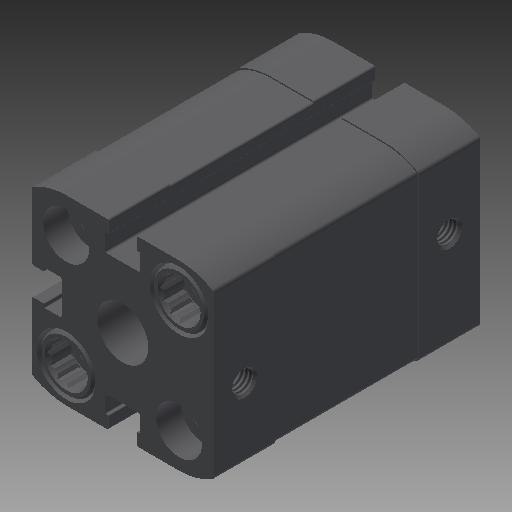
# Autodesk Inventor part: 536233 ADN-15-P---(Z)
Saved by Autodesk Inventor 2017 (Build 210142000, 142)
## iProperties
Category: PARTsolutions
Company: FESTO
Created: 2018-05-29
Part Number: 536233 ADN-15-P---(Z)
Catalog Web Link: www.cadenas.de
Description: ADN-(Z)-Compact cylinder - Z
Vendor: FESTO
Document SubType Name: Modeling
Designer: psAdmin
Manufacturer: FESTO
Mass: 44.5722 g
Surface Area: 191.377 cm^2
Volume: 44.5722 cm^3
Density: 1 g/cm^3
Material: Generic
Appearance: PSOLRGB-191-191-191
PSOL_IDENT_0: {$CADENAS_DATA\23d-libs\festo\parts\a\adn\parts\adn_zr.prj},210 {VTYP=3D},{NB=536233 ADN-15-P---(Z)}
PSOL_IDENT_1: ,{LINA=536233 ADN-15-P---(Z)},{NN=ADN-(Z)},{DATE=06.10.2015 11:54:02},{GEOMDATE=22.09.2015 09:31:00}
PSOL_IDENT_2: ,{VERSION=},{LINEID=8190},{LINESUBID=-1},{WBVAR=HUB,DF,Q,S2S20,S1,R8,TT}  {NB=536233 ADN-15-P---(Z)}
PSOL_IDENT_3: ,{LINA=536233 ADN-15-P---(Z)},{KT=536233},{TNR=536233},{AUSF=ADN},{KDM=20},{BG=19.500},{VERS=1},{HUB
PSOL_IDENT_4: P=-},{HUB=15.00000},{HUB1=[1-300]},{HUB2=[1-200]},{HUB3=0},{THC='A','I'},{DF=P},{GA=A},{HUBL=variabl
PSOL_IDENT_5: e},{HUBC=hubc error},{Q=-},{VAR1C='-','Q'},{S2S20=-},{VAR2C='-','S2','S20'},{VAR5C='-','S6'},{S1=-},
PSOL_IDENT_6: {R8=-},{R81='-','R8'},{TT=-},{TT1='-','TT'},{VAR6C='-'},{VAR7C='-','R3'},{HUBALG=[1-300]},{A=16.000}
PSOL_IDENT_7: ,{A1=0.000},{AF=14.000},{AF1=0.000},{AF2=12.000},{AF3=0.000},{B=0.000},{B1=18.000},{BG1=0.000},{D1=9
PSOL_IDENT_8: .000},{D2=9.000},{D3=4.100},{D4=0.000},{D5=6.000},{D6=M4},{D7=4.000},{D8=3.800},{D9=6.000},{E=35.500
PSOL_IDENT_9: },{EE=M5},{EEN=5.000},{EE1=-},{J=12.000},{J1=2.600},{J11=2.6},{J2=0.000},{KF=10-32 UNF-2B},{KF1=-},{
PSOL_IDENT_10: KF2=10-32 UNF-2B},{KF3=-},{KK=5/16-24 UNF-2A},{KK1=-},{L1=2.600},{L2=37.000},{L3=2.100},{L4=4.800},{
PSOL_IDENT_11: L5=0.000},{L6=51.000},{L7=17.000},{L8=2.000},{L9=2.000},{L10=0.000},{L11=0.000},{MF=8.000},{MM=10.00
PSOL_IDENT_12: 0},{MM1=0.000},{PL=6.000},{RT=M5},{RTN=5},{RTNK=4.134},{SF=11/32},{SF1=-},{SW=9.000},{TG=22.000},{VD=
PSOL_IDENT_13: 0.000},{VD1=5.200},{WH=5.700},{WH1=0.000},{WL=4.200},{WL1=0.000},{Y1=0.300},{Y2=0.500},{ZJ=42.700},{
PSOL_IDENT_14: ZM=48.400},{RU=23.800},{R1=12.750},{R2=0.800},{RA=0.000},{RB1=5.400},{RB2=6.800},{RT1=3.400},{DSK=8.
PSOL_IDENT_15: 000},{MDK=10.000},{MK=6.000},{MT=3.000},{MS=5.000},{RUB=0.400},{KFN=6.000},{KFK=4.917},{B111=11.500}
PSOL_IDENT_16: ,{B11=1.000},{B2=6.500},{B3=10.500},{B4=4.600},{B5=4.400},{B6=7.500},{B7=19.500},{B8=5.000},{B9=7.00
PSOL_IDENT_17: 0},{B10=8.400},{W=0.400},{S=7.000},{LA=0.000},{LA1=0.000},{LA2=5.500},{LA3=7.500},{LA31=11.000},{LA4=
PSOL_IDENT_18: 0.000},{LA5=0.000},{LA6=0.000},{RR=5.000},{LA7=0.000},{LA8=0.000},{LA9=0.000},{LA10=0.000},{ES=0.000
PSOL_IDENT_19: },{SS=0.000},{TS=0.000},{WS=0.000},{DK=0.000},{KS=0.000},{QN=},{S2N=},{S1S20N=},{R8N=},{TTN=},{DFALG='
PSOL_IDENT_20: P','PPS'}
NN: ADN-(Z)
NT: Compact cylinder - Z
NB: 536233 ADN-15-P---(Z)
NBSYN: $TNR. $AUSF.-$HUB.-$DF.$QN.$S2N.$S1S20N.$R8N.$TTN.---(Z)
LINA: 536233 ADN-15-P---(Z)
TNR: 536233
AUSF: ADN
KDM: 20
BG: 19.500
HUB: 15.00000
DF: P
GA: A
Q: -
S2S20: -
S1: -
R8: -
TT: -
A: 16.000
A1: 0.000
AF: 14.000
AF1: 0.000
AF2: 12.000
AF3: 0.000
B: 0.000
B1: 18.000
BG1: 0.000
D1: 9.000
D2: 9.000
D3: 4.100
D4: 0.000
D5: 6.000
D6: M4
D7: 4.000
D8: 3.800
D9: 6.000
E: 35.500
EE: M5
EE1: -
J: 12.000
J1: 2.600
J2: 0.000
KF: 10-32 UNF-2B
KF1: -
KF2: 10-32 UNF-2B
KF3: -
KK: 5/16-24 UNF-2A
KK1: -
L1: 2.600
L2: 37.000
L3: 2.100
L4: 4.800
L5: 0.000
L6: 51.000
L7: 17.000
L8: 2.000
L9: 2.000
L10: 0.000
L11: 0.000
MF: 8.000
MM: 10.000
MM1: 0.000
PL: 6.000
RT: M5
RTNK: 4.134
SF: 11/32
SF1: -
SW: 9.000
TG: 22.000
VD: 0.000
VD1: 5.200
WH: 5.700
WH1: 0.000
WL: 4.200
WL1: 0.000
Y1: 0.300
Y2: 0.500
ZJ: 42.700
ZM: 48.400
RU: 23.800
R1: 12.750
R2: 0.800
RA: 0.000
DSK: 8.000
MDK: 10.000
MK: 6.000
MT: 3.000
MS: 5.000
RUB: 0.400
B111: 11.500
B11: 1.000
B2: 6.500
B3: 10.500
B4: 4.600
B5: 4.400
B6: 7.500
B7: 19.500
B8: 5.000
B9: 7.000
B10: 8.400
W: 0.400
S: 7.000
LA: 0.000
LA1: 0.000
LA2: 5.500
LA3: 7.500
LA31: 11.000
LA4: 0.000
LA5: 0.000
LA6: 0.000
RR: 5.000
LA7: 0.000
LA8: 0.000
LA9: 0.000
LA10: 0.000
ES: 0.000
SS: 0.000
TS: 0.000
WS: 0.000
DK: 0.000
KS: 0.000
SUPPLIER: FESTO
ARTICLENO: 536233 ADN-15-P---(Z)
BOMINFO: 536233 ADN-15-P---(Z)
CREATOR: CADENAS GmbH
Title: 536233 ADN-15-P---(Z)
Author: Cadenas PARTsolutions
Comments: Compact cylinder - Z
Autodesk Inventor part; units mm, degrees
sketch "Skizze_1" plane through (0, 0, 0) normal (0, 0, 1) x (1, 0, 0)
  line L0 (-17.75, -3.1) -> (-17.75, -15.3634)
  arc A0 (-17.75, -15.3634) -> (-17.3483, -16.0572) centre (-16.95, -15.3634) ccw
  arc A1 (-17.3483, -16.0572) -> (-11, -17.75) centre (-11, -5) ccw
  line L1 (-11, -17.75) -> (-3.1, -17.75)
  arc A2 (-3.1, -17.75) -> (-2.7, -17.35) centre (-3.1, -17.35) ccw
  line L2 (-2.7, -17.35) -> (-2.7, -15.5)
  arc A3 (-2.7, -15.5) -> (-2.9, -15.3) centre (-2.9, -15.5) ccw
  line L3 (-2.9, -15.3) -> (-3.2, -15.3)
  arc A4 (-3.4, -15.1) -> (-3.2, -15.3) centre (-3.2, -15.1) ccw
  line L4 (-3.4, -15.1) -> (-3.4, -12.3)
  arc A5 (-3, -11.9) -> (-3.4, -12.3) centre (-3, -12.3) ccw
  line L5 (-3, -11.9) -> (3, -11.9)
  arc A6 (3.4, -12.3) -> (3, -11.9) centre (3, -12.3) ccw
  line L6 (3.4, -12.3) -> (3.4, -15.1)
  arc A7 (3.2, -15.3) -> (3.4, -15.1) centre (3.2, -15.1) ccw
  line L7 (3.2, -15.3) -> (2.9, -15.3)
  arc A8 (2.9, -15.3) -> (2.7, -15.5) centre (2.9, -15.5) ccw
  line L8 (2.7, -15.5) -> (2.7, -17.35)
  arc A9 (2.7, -17.35) -> (3.1, -17.75) centre (3.1, -17.35) ccw
  line L9 (3.1, -17.75) -> (11, -17.75)
  arc A10 (11, -17.75) -> (17.3483, -16.0572) centre (11, -5) ccw
  arc A11 (17.3483, -16.0572) -> (17.75, -15.3634) centre (16.95, -15.3634) ccw
  line L10 (17.75, -15.3634) -> (17.75, 15.3634)
  arc A12 (17.75, 15.3634) -> (17.3483, 16.0572) centre (16.95, 15.3634) ccw
  arc A13 (17.3483, 16.0572) -> (11, 17.75) centre (11, 5) ccw
  line L11 (11, 17.75) -> (3.1, 17.75)
  arc A14 (3.1, 17.75) -> (2.7, 17.35) centre (3.1, 17.35) ccw
  line L12 (2.7, 17.35) -> (2.7, 15.5)
  arc A15 (2.7, 15.5) -> (2.9, 15.3) centre (2.9, 15.5) ccw
  line L13 (2.9, 15.3) -> (3.2, 15.3)
  arc A16 (3.4, 15.1) -> (3.2, 15.3) centre (3.2, 15.1) ccw
  line L14 (3.4, 15.1) -> (3.4, 12.3)
  arc A17 (3, 11.9) -> (3.4, 12.3) centre (3, 12.3) ccw
  line L15 (3, 11.9) -> (-3, 11.9)
  arc A18 (-3.4, 12.3) -> (-3, 11.9) centre (-3, 12.3) ccw
  line L16 (-3.4, 12.3) -> (-3.4, 15.1)
  arc A19 (-3.2, 15.3) -> (-3.4, 15.1) centre (-3.2, 15.1) ccw
  line L17 (-3.2, 15.3) -> (-2.9, 15.3)
  arc A20 (-2.9, 15.3) -> (-2.7, 15.5) centre (-2.9, 15.5) ccw
  line L18 (-2.7, 15.5) -> (-2.7, 17.35)
  arc A21 (-2.7, 17.35) -> (-3.1, 17.75) centre (-3.1, 17.35) ccw
  line L19 (-3.1, 17.75) -> (-11, 17.75)
  arc A22 (-11, 17.75) -> (-17.3483, 16.0572) centre (-11, 5) ccw
  arc A23 (-17.3483, 16.0572) -> (-17.75, 15.3634) centre (-16.95, 15.3634) ccw
  line L20 (-17.75, 15.3634) -> (-17.75, 3.1)
  arc A24 (-17.75, 3.1) -> (-17.35, 2.7) centre (-17.35, 3.1) ccw
  line L21 (-17.35, 2.7) -> (-15.5, 2.7)
  arc A25 (-15.5, 2.7) -> (-15.3, 2.9) centre (-15.5, 2.9) ccw
  line L22 (-15.3, 2.9) -> (-15.3, 3.2)
  arc A26 (-15.1, 3.4) -> (-15.3, 3.2) centre (-15.1, 3.2) ccw
  line L23 (-15.1, 3.4) -> (-12.3, 3.4)
  arc A27 (-11.9, 3) -> (-12.3, 3.4) centre (-12.3, 3) ccw
  line L24 (-11.9, 3) -> (-11.9, -3)
  arc A28 (-12.3, -3.4) -> (-11.9, -3) centre (-12.3, -3) ccw
  line L25 (-12.3, -3.4) -> (-15.1, -3.4)
  arc A29 (-15.3, -3.2) -> (-15.1, -3.4) centre (-15.1, -3.2) ccw
  line L26 (-15.3, -3.2) -> (-15.3, -2.9)
  arc A30 (-15.3, -2.9) -> (-15.5, -2.7) centre (-15.5, -2.9) ccw
  line L27 (-15.5, -2.7) -> (-17.35, -2.7)
  arc A31 (-17.35, -2.7) -> (-17.75, -3.1) centre (-17.35, -3.1) ccw
  constraints: 64 point on circle, 56 end point, 32 centre point
extrude "Extrusion1" add sketch "Skizze_1" against normal blind 52
sketch "Sketch_111" plane through (0, 0, -12) normal (0, 0, 1) x (1, 0, 0)
  line L0 (-35.5, 35.5) -> (-35.5, -35.5)
  line L1 (-35.5, -35.5) -> (35.5, -35.5)
  line L2 (35.5, -35.5) -> (35.5, 35.5)
  line L3 (35.5, 35.5) -> (-35.5, 35.5)
  line L4 (-17.5, -3.1) -> (-17.5, -15.253)
  arc A0 (-17.5, -15.253) -> (-17.0816, -15.9561) centre (-16.7, -15.253) ccw
  arc A1 (-17.0816, -15.9561) -> (-11, -17.5) centre (-11, -4.75) ccw
  line L5 (-11, -17.5) -> (-3.1, -17.5)
  arc A2 (-3.1, -17.5) -> (-2.7, -17.1) centre (-3.1, -17.1) ccw
  line L6 (-2.7, -17.1) -> (-2.7, -15.45)
  arc A3 (-2.7, -15.45) -> (-2.85, -15.3) centre (-2.85, -15.45) ccw
  line L7 (-2.85, -15.3) -> (-3.2, -15.3)
  arc A4 (-3.4, -15.1) -> (-3.2, -15.3) centre (-3.2, -15.1) ccw
  line L8 (-3.4, -15.1) -> (-3.4, -12.3)
  arc A5 (-3, -11.9) -> (-3.4, -12.3) centre (-3, -12.3) ccw
  line L9 (-3, -11.9) -> (3, -11.9)
  arc A6 (3.4, -12.3) -> (3, -11.9) centre (3, -12.3) ccw
  line L10 (3.4, -12.3) -> (3.4, -15.1)
  arc A7 (3.2, -15.3) -> (3.4, -15.1) centre (3.2, -15.1) ccw
  line L11 (3.2, -15.3) -> (2.85, -15.3)
  arc A8 (2.85, -15.3) -> (2.7, -15.45) centre (2.85, -15.45) ccw
  line L12 (2.7, -15.45) -> (2.7, -17.1)
  arc A9 (2.7, -17.1) -> (3.1, -17.5) centre (3.1, -17.1) ccw
  line L13 (3.1, -17.5) -> (11, -17.5)
  arc A10 (11, -17.5) -> (17.0816, -15.9561) centre (11, -4.75) ccw
  arc A11 (17.0816, -15.9561) -> (17.5, -15.253) centre (16.7, -15.253) ccw
  line L14 (17.5, -15.253) -> (17.5, 15.253)
  arc A12 (17.5, 15.253) -> (17.0816, 15.9561) centre (16.7, 15.253) ccw
  arc A13 (17.0816, 15.9561) -> (11, 17.5) centre (11, 4.75) ccw
  line L15 (11, 17.5) -> (3.1, 17.5)
  arc A14 (3.1, 17.5) -> (2.7, 17.1) centre (3.1, 17.1) ccw
  line L16 (2.7, 17.1) -> (2.7, 15.45)
  arc A15 (2.7, 15.45) -> (2.85, 15.3) centre (2.85, 15.45) ccw
  line L17 (2.85, 15.3) -> (3.2, 15.3)
  arc A16 (3.4, 15.1) -> (3.2, 15.3) centre (3.2, 15.1) ccw
  line L18 (3.4, 15.1) -> (3.4, 12.3)
  arc A17 (3, 11.9) -> (3.4, 12.3) centre (3, 12.3) ccw
  line L19 (3, 11.9) -> (-3, 11.9)
  arc A18 (-3.4, 12.3) -> (-3, 11.9) centre (-3, 12.3) ccw
  line L20 (-3.4, 12.3) -> (-3.4, 15.1)
  arc A19 (-3.2, 15.3) -> (-3.4, 15.1) centre (-3.2, 15.1) ccw
  line L21 (-3.2, 15.3) -> (-2.85, 15.3)
  arc A20 (-2.85, 15.3) -> (-2.7, 15.45) centre (-2.85, 15.45) ccw
  line L22 (-2.7, 15.45) -> (-2.7, 17.1)
  arc A21 (-2.7, 17.1) -> (-3.1, 17.5) centre (-3.1, 17.1) ccw
  line L23 (-3.1, 17.5) -> (-11, 17.5)
  arc A22 (-11, 17.5) -> (-17.0816, 15.9561) centre (-11, 4.75) ccw
  arc A23 (-17.0816, 15.9561) -> (-17.5, 15.253) centre (-16.7, 15.253) ccw
  line L24 (-17.5, 15.253) -> (-17.5, 3.1)
  arc A24 (-17.5, 3.1) -> (-17.1, 2.7) centre (-17.1, 3.1) ccw
  line L25 (-17.1, 2.7) -> (-15.45, 2.7)
  arc A25 (-15.45, 2.7) -> (-15.3, 2.85) centre (-15.45, 2.85) ccw
  line L26 (-15.3, 2.85) -> (-15.3, 3.2)
  arc A26 (-15.1, 3.4) -> (-15.3, 3.2) centre (-15.1, 3.2) ccw
  line L27 (-15.1, 3.4) -> (-12.3, 3.4)
  arc A27 (-11.9, 3) -> (-12.3, 3.4) centre (-12.3, 3) ccw
  line L28 (-11.9, 3) -> (-11.9, -3)
  arc A28 (-12.3, -3.4) -> (-11.9, -3) centre (-12.3, -3) ccw
  line L29 (-12.3, -3.4) -> (-15.1, -3.4)
  arc A29 (-15.3, -3.2) -> (-15.1, -3.4) centre (-15.1, -3.2) ccw
  line L30 (-15.3, -3.2) -> (-15.3, -2.85)
  arc A30 (-15.3, -2.85) -> (-15.45, -2.7) centre (-15.45, -2.85) ccw
  line L31 (-15.45, -2.7) -> (-17.1, -2.7)
  arc A31 (-17.1, -2.7) -> (-17.5, -3.1) centre (-17.1, -3.1) ccw
  constraints: 64 end point, 64 point on circle, 32 centre point
extrude "Extrusion2" cut sketch "Sketch_111" against normal blind 28
sketch "Skizze_3_ALT_Drilling_1" plane through (0, -2.6, 0) normal (0, 1, 0) x (1, 0, 0)
  line L0 (17.75, 6) -> (10.25, 6)
  line L1 (10.25, 6) -> (10.25, 8.067)
  line L2 (10.25, 8.067) -> (17.317, 8.067)
  line L3 (17.317, 8.067) -> (17.75, 8.5)
  line L4 (17.75, 8.5) -> (17.75, 6)
  line L5 (17.75, 6) -> (10.25, 6)
  constraints: 12 end point
revolve "Revolution1" cut sketch "Skizze_3_ALT_Drilling_1" angle 360 about axis through (17.75, -2.6, -6) along (1, 0, 0)
thread "Thread1" size "M5x0.8" class "6H" standard "ISO Metric profile" length 5.067
sketch "Skizze_4_ALT_Drilling_2" plane through (0, 2.6, 0) normal (0, 1, 0) x (1, 0, 0)
  line L0 (17.75, 46) -> (6.75, 46)
  line L1 (6.75, 46) -> (6.75, 48.067)
  line L2 (6.75, 48.067) -> (17.317, 48.067)
  line L3 (17.317, 48.067) -> (17.75, 48.5)
  line L4 (17.75, 48.5) -> (17.75, 46)
  line L5 (17.75, 46) -> (6.75, 46)
  constraints: 12 end point
revolve "Revolution2" cut sketch "Skizze_4_ALT_Drilling_2" angle 360 about axis through (17.75, 2.6, -46) along (1, 0, 0)
thread "Thread2" size "M5x0.8" class "6H" standard "ISO Metric profile" length 5.067
sketch "Skizze_5_ALT_Drilling_3" plane through (0, 0, 0) normal (1, 0, 0) x (0, 1, 0)
  line L0 (0, -40) -> (0, 6.2)
  line L1 (0, 6.2) -> (5, 6.2)
  line L2 (5, 6.2) -> (5, -20)
  line L3 (5, -20) -> (10, -20)
  line L4 (10, -20) -> (10, -40)
  line L5 (10, -40) -> (0, -40)
  line L6 (0, -40) -> (0, 6.2)
  constraints: 14 end point
revolve "Revolution3" cut sketch "Skizze_5_ALT_Drilling_3" angle 360 about axis through (0, 0, -40) along (0, 0, -1)
sketch "Skizze_7_ALT_Drilling_4" plane through (0, 0, 0) normal (1, 0, 0) x (0, 1, 0)
  line L0 (0, -52) -> (0, -49.9)
  line L1 (0, -49.9) -> (4.5, -49.9)
  line L2 (4.5, -49.9) -> (4.5, -52)
  line L3 (4.5, -52) -> (0, -52)
  line L4 (0, -52) -> (0, -49.9)
  constraints: 10 end point
revolve "Revolution4" cut sketch "Skizze_7_ALT_Drilling_4" angle 360 about axis through (0, 0, -52) along (0, 0, -1)
sketch "Skizze_8_ALT_Drilling_5" plane through (11, 0, 0) normal (1, 0, 0) x (0, 0, -1)
  line L0 (19.5, 11) -> (0, 11)
  line L1 (0, 11) -> (0, 16.75)
  line L2 (0, 16.75) -> (6.5, 16.75)
  line L3 (6.5, 16.75) -> (6.5, 14.5)
  line L4 (6.5, 14.5) -> (19.5, 14.5)
  line L5 (19.5, 14.5) -> (19.5, 11)
  line L6 (19.5, 11) -> (0, 11)
  constraints: 14 end point
revolve "Revolution5" cut sketch "Skizze_8_ALT_Drilling_5" angle 360 about axis through (11, 11, -19.5) along (0, 0, -1)
sketch "Sketch_27" plane through (11, 0, 0) normal (1, 0, 0) x (0, 0, -1)
  line L0 (19.5, 11) -> (0, 11)
  line L1 (0, 15.2) -> (0.7794, 14.75)
  line L2 (0.7794, 14.75) -> (4.6, 14.75)
  line L3 (4.6, 14.75) -> (4.6, 13.5)
  line L4 (4.6, 13.5) -> (5.033, 13.067)
  line L5 (5.033, 13.067) -> (19.5, 13.067)
  line L6 (19.5, 13.067) -> (19.5, 15.5)
  line L7 (19.5, 15.5) -> (6.5, 15.5)
  line L8 (6.5, 15.5) -> (6.5, 16.25)
  line L9 (6.5, 16.25) -> (0.4, 16.25)
  line L10 (0.4, 16.25) -> (0, 15.85)
  line L11 (0, 15.85) -> (0, 15.2)
  constraints: 24 end point
revolve "Revolution6" add sketch "Sketch_27" angle 360 about axis through (11, 11, -19.5) along (0, 0, -1)
thread "Thread3" size "M5x0.8" class "6H" standard "ISO Metric profile" full length
sketch "Sketch_1_ALT_Drilling_6" plane through (11, 0, 0) normal (1, 0, 0) x (0, 0, -1)
  line L0 (52, -11) -> (32.5, -11)
  line L1 (32.5, -11) -> (32.5, -7.5)
  line L2 (32.5, -7.5) -> (45.5, -7.5)
  line L3 (45.5, -7.5) -> (45.5, -5.25)
  line L4 (45.5, -5.25) -> (52, -5.25)
  line L5 (52, -5.25) -> (52, -11)
  line L6 (52, -11) -> (32.5, -11)
  constraints: 14 end point
revolve "Revolution7" cut sketch "Sketch_1_ALT_Drilling_6" angle 360 about axis through (11, -11, -52) along (0, 0, -1)
sketch "Sketch_28" plane through (11, 0, 0) normal (1, 0, 0) x (0, 0, -1)
  line L0 (52, -11) -> (32.5, -11)
  line L1 (32.5, -6.5) -> (32.5, -8.933)
  line L2 (32.5, -8.933) -> (46.967, -8.933)
  line L3 (46.967, -8.933) -> (47.4, -8.5)
  line L4 (47.4, -8.5) -> (47.4, -7.25)
  line L5 (47.4, -7.25) -> (51.2206, -7.25)
  line L6 (51.2206, -7.25) -> (52, -6.8)
  line L7 (52, -6.8) -> (52, -6.15)
  line L8 (52, -6.15) -> (51.6, -5.75)
  line L9 (51.6, -5.75) -> (45.5, -5.75)
  line L10 (45.5, -5.75) -> (45.5, -6.5)
  line L11 (45.5, -6.5) -> (32.5, -6.5)
  constraints: 24 end point
revolve "Revolution8" add sketch "Sketch_28" angle 360 about axis through (11, -11, -52) along (0, 0, -1)
thread "Thread4" size "M5x0.8" class "6H" standard "ISO Metric profile" full length
sketch "Skizze_9_ALT_Drilling_7" plane through (-11, 0, 0) normal (1, 0, 0) x (0, 0, -1)
  line L0 (26, -11) -> (0, -11)
  line L1 (0, -11) -> (0, -5.25)
  line L2 (0, -5.25) -> (6.5, -5.25)
  line L3 (6.5, -5.25) -> (6.5, -7.5)
  line L4 (6.5, -7.5) -> (19.5, -7.5)
  line L5 (19.5, -7.5) -> (19.5, -11)
  line L6 (19.5, -11) -> (0, -11)
  constraints: 14 end point
revolve "Revolution9" cut sketch "Skizze_9_ALT_Drilling_7" angle 360 about axis through (-11, -11, -26) along (0, 0, -1)
sketch "Sketch_2_ALT_Drilling_8" plane through (-11, 0, 0) normal (1, 0, 0) x (0, 0, -1)
  line L0 (52, 11) -> (32.5, 11)
  line L1 (32.5, 11) -> (32.5, 14.5)
  line L2 (32.5, 14.5) -> (45.5, 14.5)
  line L3 (45.5, 14.5) -> (45.5, 16.75)
  line L4 (45.5, 16.75) -> (52, 16.75)
  line L5 (52, 16.75) -> (52, 11)
  line L6 (52, 11) -> (32.5, 11)
  constraints: 14 end point
revolve "Revolution10" cut sketch "Sketch_2_ALT_Drilling_8" angle 360 about axis through (-11, 11, -52) along (0, 0, -1)
sketch "Sketch_29" plane through (-11, 0, 0) normal (1, 0, 0) x (0, 0, -1)
  line L0 (19.5, -11) -> (0, -11)
  line L1 (0, -6.8) -> (0.7794, -7.25)
  line L2 (0.7794, -7.25) -> (4.6, -7.25)
  line L3 (4.6, -7.25) -> (4.6, -8.5)
  line L4 (4.6, -8.5) -> (5.033, -8.933)
  line L5 (5.033, -8.933) -> (19.5, -8.933)
  line L6 (19.5, -8.933) -> (19.5, -6.5)
  line L7 (19.5, -6.5) -> (6.5, -6.5)
  line L8 (6.5, -6.5) -> (6.5, -5.75)
  line L9 (6.5, -5.75) -> (0.4, -5.75)
  line L10 (0.4, -5.75) -> (0, -6.15)
  line L11 (0, -6.15) -> (0, -6.8)
  constraints: 24 end point
revolve "Revolution11" add sketch "Sketch_29" angle 360 about axis through (-11, -11, -19.5) along (0, 0, -1)
thread "Thread5" size "M5x0.8" class "6H" standard "ISO Metric profile" full length
sketch "Sketch_30" plane through (-11, 0, 0) normal (1, 0, 0) x (0, 0, -1)
  line L0 (52, 11) -> (32.5, 11)
  line L1 (32.5, 15.5) -> (32.5, 13.067)
  line L2 (32.5, 13.067) -> (46.967, 13.067)
  line L3 (46.967, 13.067) -> (47.4, 13.5)
  line L4 (47.4, 13.5) -> (47.4, 14.75)
  line L5 (47.4, 14.75) -> (51.2206, 14.75)
  line L6 (51.2206, 14.75) -> (52, 15.2)
  line L7 (52, 15.2) -> (52, 15.85)
  line L8 (52, 15.85) -> (51.6, 16.25)
  line L9 (51.6, 16.25) -> (45.5, 16.25)
  line L10 (45.5, 16.25) -> (45.5, 15.5)
  line L11 (45.5, 15.5) -> (32.5, 15.5)
  constraints: 24 end point
revolve "Revolution12" add sketch "Sketch_30" angle 360 about axis through (-11, 11, -52) along (0, 0, -1)
thread "Thread6" size "M5x0.8" class "6H" standard "ISO Metric profile" full length
sketch "Skizze_12_ALT_Drilling_9" plane through (11, 0, 0) normal (1, 0, 0) x (0, 0, -1)
  line L0 (32.5, -11) -> (-0.1, -11)
  line L1 (-0.1, -11) -> (-0.1, -6.5)
  line L2 (-0.1, -6.5) -> (4.8, -6.5)
  line L3 (4.8, -6.5) -> (4.8, -8.5)
  line L4 (4.8, -8.5) -> (5.233, -8.933)
  line L5 (5.233, -8.933) -> (32.5, -8.933)
  line L6 (32.5, -8.933) -> (32.5, -11)
  line L7 (32.5, -11) -> (-0.1, -11)
  constraints: 16 end point
revolve "Revolution13" cut sketch "Skizze_12_ALT_Drilling_9" angle 360 about axis through (11, -11, -32.5) along (0, 0, -1)
thread "Thread7" size "M5x0.8" class "6H" standard "ISO Metric profile" length 6.767
sketch "Sketch_123" plane through (11, 0, 0) normal (1, 0, 0) x (0, 0, -1)
  line L0 (32.5, -11) -> (12, -11)
  line L1 (12, -11) -> (12, -6.5)
  line L2 (12, -6.5) -> (32.5, -6.5)
  line L3 (32.5, -6.5) -> (32.5, -11)
  line L4 (32.5, -11) -> (12, -11)
  constraints: 10 end point
revolve "Revolution14" add sketch "Sketch_123" angle 360 about axis through (11, -11, -32.5) along (0, 0, -1)
sketch "Sketch_124_ALT_Drilling_10" plane through (11, 0, 0) normal (1, 0, 0) x (0, 0, -1)
  line L0 (32.5, -11) -> (12, -11)
  line L1 (12, -11) -> (12, -8.5)
  line L2 (12, -8.5) -> (32.5, -8.5)
  line L3 (32.5, -8.5) -> (32.5, -11)
  line L4 (32.5, -11) -> (12, -11)
  constraints: 10 end point
revolve "Revolution15" cut sketch "Sketch_124_ALT_Drilling_10" angle 360 about axis through (11, -11, -32.5) along (0, 0, -1)
sketch "Sketch_3_ALT_Drilling_11" plane through (11, 0, 0) normal (1, 0, 0) x (0, 0, -1)
  line L0 (52.1, 11) -> (26, 11)
  line L1 (26, 11) -> (26, 13.067)
  line L2 (26, 13.067) -> (46.767, 13.067)
  line L3 (46.767, 13.067) -> (47.2, 13.5)
  line L4 (47.2, 13.5) -> (47.2, 15.5)
  line L5 (47.2, 15.5) -> (52.1, 15.5)
  line L6 (52.1, 15.5) -> (52.1, 11)
  line L7 (52.1, 11) -> (26, 11)
  constraints: 16 end point
revolve "Revolution16" cut sketch "Sketch_3_ALT_Drilling_11" angle 360 about axis through (11, 11, -52.1) along (0, 0, -1)
thread "Thread8" size "M5x0.8" class "6H" standard "ISO Metric profile" length 6.767
sketch "Sketch_117" plane through (11, 0, 0) normal (1, 0, 0) x (0, 0, -1)
  line L0 (40, 11) -> (19.5, 11)
  line L1 (19.5, 11) -> (19.5, 15.5)
  line L2 (19.5, 15.5) -> (40, 15.5)
  line L3 (40, 15.5) -> (40, 11)
  line L4 (40, 11) -> (19.5, 11)
  constraints: 10 end point
revolve "Revolution17" add sketch "Sketch_117" angle 360 about axis through (11, 11, -40) along (0, 0, -1)
sketch "Sketch_119_ALT_Drilling_12" plane through (11, 0, 0) normal (1, 0, 0) x (0, 0, -1)
  line L0 (40, 11) -> (19.5, 11)
  line L1 (19.5, 11) -> (19.5, 13.5)
  line L2 (19.5, 13.5) -> (40, 13.5)
  line L3 (40, 13.5) -> (40, 11)
  line L4 (40, 11) -> (19.5, 11)
  constraints: 10 end point
revolve "Revolution18" cut sketch "Sketch_119_ALT_Drilling_12" angle 360 about axis through (11, 11, -40) along (0, 0, -1)
sketch "Skizze_13_ALT_Drilling_13" plane through (-11, 0, 0) normal (1, 0, 0) x (0, 0, -1)
  line L0 (32.5, 11) -> (-0.1, 11)
  line L1 (-0.1, 11) -> (-0.1, 15.5)
  line L2 (-0.1, 15.5) -> (4.8, 15.5)
  line L3 (4.8, 15.5) -> (4.8, 13.5)
  line L4 (4.8, 13.5) -> (5.233, 13.067)
  line L5 (5.233, 13.067) -> (32.5, 13.067)
  line L6 (32.5, 13.067) -> (32.5, 11)
  line L7 (32.5, 11) -> (-0.1, 11)
  constraints: 16 end point
revolve "Revolution19" cut sketch "Skizze_13_ALT_Drilling_13" angle 360 about axis through (-11, 11, -32.5) along (0, 0, -1)
thread "Thread9" size "M5x0.8" class "6H" standard "ISO Metric profile" length 6.767
sketch "Sketch_121" plane through (-11, 0, 0) normal (1, 0, 0) x (0, 0, -1)
  line L0 (32.5, 11) -> (12, 11)
  line L1 (12, 11) -> (12, 15.5)
  line L2 (12, 15.5) -> (32.5, 15.5)
  line L3 (32.5, 15.5) -> (32.5, 11)
  line L4 (32.5, 11) -> (12, 11)
  constraints: 10 end point
revolve "Revolution20" add sketch "Sketch_121" angle 360 about axis through (-11, 11, -32.5) along (0, 0, -1)
sketch "Sketch_122_ALT_Drilling_14" plane through (-11, 0, 0) normal (1, 0, 0) x (0, 0, -1)
  line L0 (32.5, 11) -> (12, 11)
  line L1 (12, 11) -> (12, 13.5)
  line L2 (12, 13.5) -> (32.5, 13.5)
  line L3 (32.5, 13.5) -> (32.5, 11)
  line L4 (32.5, 11) -> (12, 11)
  constraints: 10 end point
revolve "Revolution21" cut sketch "Sketch_122_ALT_Drilling_14" angle 360 about axis through (-11, 11, -32.5) along (0, 0, -1)
sketch "Sketch_4_ALT_Drilling_15" plane through (-11, 0, 0) normal (1, 0, 0) x (0, 0, -1)
  line L0 (52.1, -11) -> (26, -11)
  line L1 (26, -11) -> (26, -8.933)
  line L2 (26, -8.933) -> (46.767, -8.933)
  line L3 (46.767, -8.933) -> (47.2, -8.5)
  line L4 (47.2, -8.5) -> (47.2, -6.5)
  line L5 (47.2, -6.5) -> (52.1, -6.5)
  line L6 (52.1, -6.5) -> (52.1, -11)
  line L7 (52.1, -11) -> (26, -11)
  constraints: 16 end point
revolve "Revolution22" cut sketch "Sketch_4_ALT_Drilling_15" angle 360 about axis through (-11, -11, -52.1) along (0, 0, -1)
thread "Thread10" size "M5x0.8" class "6H" standard "ISO Metric profile" length 6.767
sketch "Sketch_118" plane through (-11, 0, 0) normal (1, 0, 0) x (0, 0, -1)
  line L0 (40, -11) -> (19.5, -11)
  line L1 (19.5, -11) -> (19.5, -6.5)
  line L2 (19.5, -6.5) -> (40, -6.5)
  line L3 (40, -6.5) -> (40, -11)
  line L4 (40, -11) -> (19.5, -11)
  constraints: 10 end point
revolve "Revolution23" add sketch "Sketch_118" angle 360 about axis through (-11, -11, -40) along (0, 0, -1)
sketch "Sketch_120_ALT_Drilling_16" plane through (-11, 0, 0) normal (1, 0, 0) x (0, 0, -1)
  line L0 (40, -11) -> (19.5, -11)
  line L1 (19.5, -11) -> (19.5, -8.5)
  line L2 (19.5, -8.5) -> (40, -8.5)
  line L3 (40, -8.5) -> (40, -11)
  line L4 (40, -11) -> (19.5, -11)
  constraints: 10 end point
revolve "Revolution24" cut sketch "Sketch_120_ALT_Drilling_16" angle 360 about axis through (-11, -11, -40) along (0, 0, -1)
sketch "Sketch_8" plane through (0, 0, 0) normal (0, 0, 1) x (1, 0, 0)
  line L0 (-15.0415, -11) -> (-14.5, -11.9378)
  line L1 (-14.5, -11.9378) -> (-14.5, -13.0207)
  line L2 (-14.5, -13.0207) -> (-13.5622, -13.5622)
  line L3 (-13.5622, -13.5622) -> (-13.0207, -14.5)
  line L4 (-13.0207, -14.5) -> (-11.9378, -14.5)
  line L5 (-11.9378, -14.5) -> (-11, -15.0415)
  line L6 (-11, -15.0415) -> (-10.0622, -14.5)
  line L7 (-10.0622, -14.5) -> (-8.9793, -14.5)
  line L8 (-8.9793, -14.5) -> (-8.4378, -13.5622)
  line L9 (-8.4378, -13.5622) -> (-7.5, -13.0207)
  line L10 (-7.5, -13.0207) -> (-7.5, -11.9378)
  line L11 (-7.5, -11.9378) -> (-6.9585, -11)
  line L12 (-6.9585, -11) -> (-7.5, -10.0622)
  line L13 (-7.5, -10.0622) -> (-7.5, -8.9793)
  line L14 (-7.5, -8.9793) -> (-8.4378, -8.4378)
  line L15 (-8.4378, -8.4378) -> (-8.9793, -7.5)
  line L16 (-8.9793, -7.5) -> (-10.0622, -7.5)
  line L17 (-10.0622, -7.5) -> (-11, -6.9585)
  line L18 (-11, -6.9585) -> (-11.9378, -7.5)
  line L19 (-11.9378, -7.5) -> (-13.0207, -7.5)
  line L20 (-13.0207, -7.5) -> (-13.5622, -8.4378)
  line L21 (-13.5622, -8.4378) -> (-14.5, -8.9793)
  line L22 (-14.5, -8.9793) -> (-14.5, -10.0622)
  line L23 (-14.5, -10.0622) -> (-15.0415, -11)
  constraints: 48 end point
extrude "Extrusion3" cut sketch "Sketch_8" against normal blind 4.4
sketch "Sketch_7" plane through (0, 0, 0) normal (0, 0, 1) x (1, 0, 0)
  line L0 (6.9585, 11) -> (7.5, 10.0622)
  line L1 (7.5, 10.0622) -> (7.5, 8.9793)
  line L2 (7.5, 8.9793) -> (8.4378, 8.4378)
  line L3 (8.4378, 8.4378) -> (8.9793, 7.5)
  line L4 (8.9793, 7.5) -> (10.0622, 7.5)
  line L5 (10.0622, 7.5) -> (11, 6.9585)
  line L6 (11, 6.9585) -> (11.9378, 7.5)
  line L7 (11.9378, 7.5) -> (13.0207, 7.5)
  line L8 (13.0207, 7.5) -> (13.5622, 8.4378)
  line L9 (13.5622, 8.4378) -> (14.5, 8.9793)
  line L10 (14.5, 8.9793) -> (14.5, 10.0622)
  line L11 (14.5, 10.0622) -> (15.0415, 11)
  line L12 (15.0415, 11) -> (14.5, 11.9378)
  line L13 (14.5, 11.9378) -> (14.5, 13.0207)
  line L14 (14.5, 13.0207) -> (13.5622, 13.5622)
  line L15 (13.5622, 13.5622) -> (13.0207, 14.5)
  line L16 (13.0207, 14.5) -> (11.9378, 14.5)
  line L17 (11.9378, 14.5) -> (11, 15.0415)
  line L18 (11, 15.0415) -> (10.0622, 14.5)
  line L19 (10.0622, 14.5) -> (8.9793, 14.5)
  line L20 (8.9793, 14.5) -> (8.4378, 13.5622)
  line L21 (8.4378, 13.5622) -> (7.5, 13.0207)
  line L22 (7.5, 13.0207) -> (7.5, 11.9378)
  line L23 (7.5, 11.9378) -> (6.9585, 11)
  constraints: 48 end point
extrude "Extrusion4" cut sketch "Sketch_7" against normal blind 4.4
sketch "Sketch_9" plane through (0, 0, -52) normal (0, 0, 1) x (1, 0, 0)
  line L0 (-15.0415, 11) -> (-14.5, 10.0622)
  line L1 (-14.5, 10.0622) -> (-14.5, 8.9793)
  line L2 (-14.5, 8.9793) -> (-13.5622, 8.4378)
  line L3 (-13.5622, 8.4378) -> (-13.0207, 7.5)
  line L4 (-13.0207, 7.5) -> (-11.9378, 7.5)
  line L5 (-11.9378, 7.5) -> (-11, 6.9585)
  line L6 (-11, 6.9585) -> (-10.0622, 7.5)
  line L7 (-10.0622, 7.5) -> (-8.9793, 7.5)
  line L8 (-8.9793, 7.5) -> (-8.4378, 8.4378)
  line L9 (-8.4378, 8.4378) -> (-7.5, 8.9793)
  line L10 (-7.5, 8.9793) -> (-7.5, 10.0622)
  line L11 (-7.5, 10.0622) -> (-6.9585, 11)
  line L12 (-6.9585, 11) -> (-7.5, 11.9378)
  line L13 (-7.5, 11.9378) -> (-7.5, 13.0207)
  line L14 (-7.5, 13.0207) -> (-8.4378, 13.5622)
  line L15 (-8.4378, 13.5622) -> (-8.9793, 14.5)
  line L16 (-8.9793, 14.5) -> (-10.0622, 14.5)
  line L17 (-10.0622, 14.5) -> (-11, 15.0415)
  line L18 (-11, 15.0415) -> (-11.9378, 14.5)
  line L19 (-11.9378, 14.5) -> (-13.0207, 14.5)
  line L20 (-13.0207, 14.5) -> (-13.5622, 13.5622)
  line L21 (-13.5622, 13.5622) -> (-14.5, 13.0207)
  line L22 (-14.5, 13.0207) -> (-14.5, 11.9378)
  line L23 (-14.5, 11.9378) -> (-15.0415, 11)
  constraints: 48 end point
extrude "Extrusion5" cut sketch "Sketch_9" along normal blind 4.4
sketch "Sketch_10" plane through (0, 0, -52) normal (0, 0, 1) x (1, 0, 0)
  line L0 (6.9585, -11) -> (7.5, -11.9378)
  line L1 (7.5, -11.9378) -> (7.5, -13.0207)
  line L2 (7.5, -13.0207) -> (8.4378, -13.5622)
  line L3 (8.4378, -13.5622) -> (8.9793, -14.5)
  line L4 (8.9793, -14.5) -> (10.0622, -14.5)
  line L5 (10.0622, -14.5) -> (11, -15.0415)
  line L6 (11, -15.0415) -> (11.9378, -14.5)
  line L7 (11.9378, -14.5) -> (13.0207, -14.5)
  line L8 (13.0207, -14.5) -> (13.5622, -13.5622)
  line L9 (13.5622, -13.5622) -> (14.5, -13.0207)
  line L10 (14.5, -13.0207) -> (14.5, -11.9378)
  line L11 (14.5, -11.9378) -> (15.0415, -11)
  line L12 (15.0415, -11) -> (14.5, -10.0622)
  line L13 (14.5, -10.0622) -> (14.5, -8.9793)
  line L14 (14.5, -8.9793) -> (13.5622, -8.4378)
  line L15 (13.5622, -8.4378) -> (13.0207, -7.5)
  line L16 (13.0207, -7.5) -> (11.9378, -7.5)
  line L17 (11.9378, -7.5) -> (11, -6.9585)
  line L18 (11, -6.9585) -> (10.0622, -7.5)
  line L19 (10.0622, -7.5) -> (8.9793, -7.5)
  line L20 (8.9793, -7.5) -> (8.4378, -8.4378)
  line L21 (8.4378, -8.4378) -> (7.5, -8.9793)
  line L22 (7.5, -8.9793) -> (7.5, -10.0622)
  line L23 (7.5, -10.0622) -> (6.9585, -11)
  constraints: 48 end point
extrude "Extrusion6" cut sketch "Sketch_10" along normal blind 4.4
ref_plane "CYLINDER_XY" through (0, 0, -40) normal (0, 0, 1) x (1, 0, 0)
ref_plane "CYLINDER_YZ" through (0, 0, -40) normal (1, 0, 0) x (0, 1, 0)
ref_plane "CYLINDER_ZX" through (0, 0, -40) normal (0, 1, 0) x (0, 0, 1)
ref_plane "FDT_FRONT_XY" through (0, 0, 0) normal (0, 0, 1) x (0, -1, 0)
ref_plane "FDT_FRONT_YZ" through (0, 0, 0) normal (0, -1, 0) x (1, 0, 0)
ref_plane "FDT_FRONT_ZX" through (0, 0, 0) normal (1, 0, 0) x (0, 0, 1)
ref_plane "FDT_QSFRONT_XY" through (17.75, -2.6, -6) normal (1, 0, 0) x (0, -1, 0)
ref_plane "FDT_QSFRONT_YZ" through (17.75, -2.6, -6) normal (0, -1, 0) x (0, 0, -1)
ref_plane "FDT_QSFRONT_ZX" through (17.75, -2.6, -6) normal (0, 0, -1) x (1, 0, 0)
ref_plane "FDT_QSREAR_XY" through (17.75, 2.6, -46) normal (1, 0, 0) x (0, -1, 0)
ref_plane "FDT_QSREAR_YZ" through (17.75, 2.6, -46) normal (0, -1, 0) x (0, 0, -1)
ref_plane "FDT_QSREAR_ZX" through (17.75, 2.6, -46) normal (0, 0, -1) x (1, 0, 0)
ref_plane "FDT_REAR_XY" through (0, 0, -52) normal (0, 0, 1) x (0, -1, 0)
ref_plane "FDT_REAR_YZ" through (0, 0, -52) normal (0, -1, 0) x (1, 0, 0)
ref_plane "FDT_REAR_ZX" through (0, 0, -52) normal (1, 0, 0) x (0, 0, 1)
ref_plane "FDT_SLOT3_1_XY" through (0, 11.9, -26) normal (0, 1, 0) x (1, 0, 0)
ref_plane "FDT_SLOT3_1_YZ" through (0, 11.9, -26) normal (1, 0, 0) x (0, 0, -1)
ref_plane "FDT_SLOT3_1_ZX" through (0, 11.9, -26) normal (0, 0, -1) x (0, 1, 0)
ref_plane "FDT_SLOT5_1_XY" through (-11.9, 0, -26) normal (-1, 0, 0) x (0, 1, 0)
ref_plane "FDT_SLOT5_1_YZ" through (-11.9, 0, -26) normal (0, 1, 0) x (0, 0, -1)
ref_plane "FDT_SLOT5_1_ZX" through (-11.9, 0, -26) normal (0, 0, -1) x (-1, 0, 0)
ref_plane "FDT_SLOT7_1_XY" through (0, -11.9, -26) normal (0, -1, 0) x (-1, 0, 0)
ref_plane "FDT_SLOT7_1_YZ" through (0, -11.9, -26) normal (-1, 0, 0) x (0, 0, -1)
ref_plane "FDT_SLOT7_1_ZX" through (0, -11.9, -26) normal (0, 0, -1) x (0, -1, 0)
ref_plane "TO_DUMMY_XY" through (0, 0, 0) normal (0, 0, 1) x (1, 0, 0)
ref_plane "TO_DUMMY_YZ" through (0, 0, 0) normal (1, 0, 0) x (0, 1, 0)
ref_plane "TO_DUMMY_ZX" through (0, 0, 0) normal (0, 1, 0) x (0, 0, 1)
body "Solid1"
